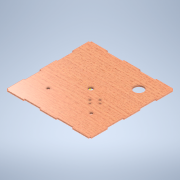
# Autodesk Inventor part: FloorPlateTop_V2
Saved by Autodesk Inventor 2022.2 (Build 262287000, 287)
## iProperties
Created: 2022-11-22
Part Number: FloorPlateTop_V2
Material: Wood (Oak)
Document SubType Name: Modeling
Designer: jaege
Density: 0.76 g/cm^3
Appearance: Red Oak - Natural Low Gloss
Mass: 194.146 g
Surface Area: 1331.73 cm^2
Volume: 255.456 cm^3
Author: jaege
Autodesk Inventor part; units mm, degrees
ref_plane "YZ Plane" through (0, 0, 0) normal (1, 0, 0) x (0, 1, 0)
ref_plane "XZ Plane" through (0, 0, 0) normal (0, 1, 0) x (-1, 0, 0)
ref_plane "XY Plane" through (0, 0, 0) normal (0, 0, 1) x (1, 0, 0)
sketch "Sketch1" plane through (0, 0, 0) normal (0, 1, 0) x (-1, 0, 0)
  line L0 (-125, 125) -> (125, 125)
  line L1 (125, 125) -> (125, -125)
  line L2 (125, -125) -> (-125, -125)
  line L3 (-125, -125) -> (-125, 125)
  line L4 (-125, 125) -> (125, -125) construction
  line L5 (125, 125) -> (-125, -125) construction
  line L6 (125, -125) -> (75, -125)
  line L7 (75, -125) -> (75, -129)
  line L8 (75, -129) -> (125, -129)
  line L9 (125, -129) -> (125, -125)
  line L10 (125, -125) -> (129, -125)
  line L11 (129, -125) -> (129, -75)
  line L12 (129, -75) -> (125, -75)
  line L13 (125, -75) -> (125, -125)
  line L14 (-125, -125) -> (-129, -125)
  line L15 (-129, -125) -> (-129, -75)
  line L16 (-129, -75) -> (-125, -75)
  line L17 (-125, -75) -> (-125, -125)
  line L18 (125, 125) -> (75, 125)
  line L19 (75, 125) -> (75, 129)
  line L20 (75, 129) -> (125, 129)
  line L21 (125, 129) -> (125, 125)
  line L22 (75, -129) -> (75, -125)
  line L23 (75, -125) -> (25, -125)
  line L24 (25, -125) -> (25, -129)
  line L25 (25, -129) -> (75, -129)
  line L26 (25, -129) -> (25, -125)
  line L27 (25, -125) -> (-25, -125)
  line L28 (-25, -125) -> (-25, -129)
  line L29 (-25, -129) -> (25, -129)
  line L30 (-25, -129) -> (-25, -125)
  line L31 (-25, -125) -> (-75, -125)
  line L32 (-75, -125) -> (-75, -129)
  line L33 (-75, -129) -> (-25, -129)
  line L34 (-75, -129) -> (-75, -125)
  line L35 (-75, -125) -> (-125, -125)
  line L36 (-125, -125) -> (-125, -129)
  line L37 (-125, -129) -> (-75, -129)
  line L38 (125, -75) -> (129, -75)
  line L39 (125, -25) -> (125, -75)
  line L40 (129, -25) -> (125, -25)
  line L41 (129, -75) -> (129, -25)
  line L42 (125, -25) -> (129, -25)
  line L43 (125, 25) -> (125, -25)
  line L44 (129, 25) -> (125, 25)
  line L45 (129, -25) -> (129, 25)
  line L46 (125, 25) -> (129, 25)
  line L47 (125, 75) -> (125, 25)
  line L48 (129, 75) -> (125, 75)
  line L49 (129, 25) -> (129, 75)
  line L50 (125, 75) -> (129, 75)
  line L51 (125, 125) -> (125, 75)
  line L52 (129, 125) -> (125, 125)
  line L53 (129, 75) -> (129, 125)
  line L54 (-125, -75) -> (-129, -75)
  line L55 (-129, -75) -> (-129, -25)
  line L56 (-129, -25) -> (-125, -25)
  line L57 (-125, -25) -> (-125, -75)
  line L58 (-125, -25) -> (-129, -25)
  line L59 (-129, -25) -> (-129, 25)
  line L60 (-129, 25) -> (-125, 25)
  line L61 (-125, 25) -> (-125, -25)
  line L62 (-125, 25) -> (-129, 25)
  line L63 (-129, 25) -> (-129, 75)
  line L64 (-129, 75) -> (-125, 75)
  line L65 (-125, 75) -> (-125, 25)
  line L66 (-125, 75) -> (-129, 75)
  line L67 (-129, 75) -> (-129, 125)
  line L68 (-129, 125) -> (-125, 125)
  line L69 (-125, 125) -> (-125, 75)
  line L70 (75, 125) -> (25, 125)
  line L71 (25, 125) -> (25, 129)
  line L72 (25, 129) -> (75, 129)
  line L73 (75, 129) -> (75, 125)
  line L74 (25, 125) -> (-25, 125)
  line L75 (-25, 125) -> (-25, 129)
  line L76 (-25, 129) -> (25, 129)
  line L77 (25, 129) -> (25, 125)
  line L78 (-25, 125) -> (-75, 125)
  line L79 (-75, 125) -> (-75, 129)
  line L80 (-75, 129) -> (-25, 129)
  line L81 (-25, 129) -> (-25, 125)
  line L82 (-75, 125) -> (-125, 125)
  line L83 (-125, 125) -> (-125, 129)
  line L84 (-125, 129) -> (-75, 129)
  line L85 (-75, 129) -> (-75, 125)
  point P0 (0, 0)
  dimension "d0" = 250
  dimension "d1" = 250
  dimension "d2" = 50
  dimension "d3" = 4
  dimension "d4" = 4
  dimension "d5" = 50
  dimension "d6" = 4
  dimension "d7" = 50
  dimension "d8" = 50
  dimension "d9" = 4
  dimension "d12" = 50
  dimension "d19" = 50
  dimension "d26" = 50
  dimension "d33" = 50
  constraints: 172 end point, 10 parallel, 7 horizontal, 5 perpendicular, 2 midpoint, 2 vertical, 136 other
  measures "d0" distance of L1.end L2.end
  measures "d1" distance of L0.end L1.end
  measures "d2" distance of L8.end L7.end
  measures "d3" distance of L7.end L6.end
  measures "d4" distance of L12.end L11.end
  measures "d5" distance of L11.end L10.end
  measures "d6" distance of L15.end L16.end
  measures "d7" distance of L14.end L15.end
  measures "d8" distance of L19.end L20.end
  measures "d9" distance of L18.end L19.end
  measures "d12" distance of L1.end L22.end
  measures "d19" distance of L1.end L38.start
  measures "d26" distance of L2.end L54.start
  measures "d33" distance of L0.end L70.start
extrude "Extrusion1" add sketch "Sketch1" along normal blind 4 contours L83 L84 L79 L0 | L0 L1 L2 L3 | L3 L64 L67 L68 | L75 L76 L71 L0 | L3 L56 L59 L60 | L19 L20 L21 L0 | L3 L14 L15 L16 | L52 L53 L48 L1 | L2 L32 L37 L36 | L44 L45 L40 L1 | L2 L24 L29 L28 | L12 L11 L10 L1 | L2 L9 L8 L7
sketch "Sketch2" plane through (0, 4, 0) normal (0, 1, 0) x (1, 0, 0)
  line L0 (25, -125) -> (75, -125) construction
  circle A0 centre (0, 2.3) radius 6.5
  circle A1 centre (-66, -62.2) radius 4
  circle A2 centre (66, -62.2) radius 4
  line L1 (0, 180.6) -> (0, -180.6) construction
  line L2 (-93.2324, -124) -> (95.467, -124) construction
  line L3 (-129, -125) -> (-125, -125) projected
  line L4 (25, -29.4721) -> (29.2426, -25.2294)
  line L5 (44.799, -9.6731) -> (47.6274, -12.5015)
  line L6 (47.6274, -12.5015) -> (43.3848, -16.7442)
  line L7 (27.8284, -32.3005) -> (25, -29.4721)
  line L8 (34.8995, -39.3716) -> (39.1421, -35.1289)
  line L9 (54.6985, -19.5726) -> (57.5269, -22.401)
  line L10 (57.5269, -22.401) -> (53.2843, -26.6437)
  line L11 (37.7279, -42.2) -> (34.8995, -39.3716)
  line L12 (40.5563, -13.9157) -> (43.3848, -16.7442)
  line L13 (29.2426, -25.2294) -> (32.0711, -28.0579)
  line L14 (39.1421, -35.1289) -> (41.9706, -37.9574)
  line L15 (50.4558, -23.8152) -> (53.2843, -26.6437)
  line L16 (40.5563, -13.9157) -> (44.799, -9.6731)
  line L17 (29.2426, -25.2294) -> (40.5563, -13.9157) construction
  line L18 (43.3848, -16.7442) -> (32.0711, -28.0579) construction
  line L19 (50.4558, -23.8152) -> (54.6985, -19.5726)
  line L20 (53.2843, -26.6437) -> (41.9706, -37.9574) construction
  line L21 (32.0711, -28.0579) -> (27.8284, -32.3005)
  line L22 (39.1421, -35.1289) -> (50.4558, -23.8152) construction
  line L23 (41.9706, -37.9574) -> (37.7279, -42.2)
  point P0 (0, 0)
  point P1 (26.4142, -30.8863)
  dimension "d46" = 13
  dimension "d52" = 8
  dimension "d53" = 132
  dimension "d54" = 61.8
  dimension "d55" = 1
  dimension "d56" = 64.5
  dimension "d57" = 10
  dimension "d58" = 4
  dimension "d59" = 6
  dimension "d60" = 6
  dimension "d61" = 45
  dimension "d62" = 20
  dimension "d63" = 28
  dimension "d64" = 25
  constraints: 42 end point, 20 parallel, 15 perpendicular, 6 point on line, 3 centre point, 3 collinear, 1 equal radius, 1 horizontal, 1 horizontal alignment, 1 midpoint, 1 symmetric about line, 1 vertical alignment
  measures "d46" diameter of A0
  measures "d52" diameter of A1
  measures "d53" distance of A2.centre A1.centre
  measures "d54" distance from line of A2.centre L2
  measures "d55" distance between parallel lines of L3 L2
  measures "d56" vertical distance of A1.centre A0.centre
  measures "d57" distance between parallel lines of L8 L6
  measures "d58" distance of L5.start L5.end
  measures "d59" distance of L5.start L12.start
  measures "d60" distance from line of point (26.414, -30.886) L13
  measures "d61" angle of L1 L4
  measures "d62" vertical distance of A2.centre L11.start
  measures "d63" distance of L9.end L11.start
  measures "d64" distance from line of L1 L4.start
extrude "Extrusion2" cut sketch "Sketch2" against normal up to next
sketch "Sketch3" plane through (0, 4, 0) normal (0, 1, 0) x (1, 0, 0)
  point P0 (0, 0)
sketch "Sketch4" plane through (0, 4, 0) normal (0, 1, 0) x (1, 0, 0)
  circle A0 centre (75, 75) radius 15
  line L0 (75, 125) -> (25, 125) projected
  line L1 (125, 25) -> (125, 75) projected
  point P0 (0, 0)
  dimension "d65" = 30
  dimension "d66" = 50
  dimension "d67" = 50
  constraints: 1 centre point
  measures "d65" diameter of A0
  measures "d66" distance from line of A0.centre L0
  measures "d67" distance from line of L1 A0.centre
extrude "Extrusion3" cut sketch "Sketch4" against normal blind 10
body "Solid1"
